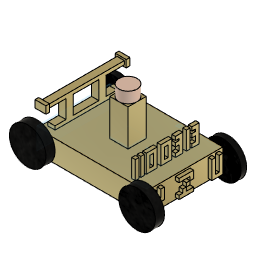
final_project_1100313 (Autodesk Fusion 360 design; units mm, degrees)
Autodesk Fusion 360 part; units mm, degrees
note: some values were not read from the file. Chosen so that the rebuilt part matches the saved one: which face or edge a step refers to; that a step has no effect; which bodies a step acts on; which pieces of a blend or face edit are solid.
(part 1 of 2)
sketch "Sketch1" plane through (0, 0, 0) normal (0, 0, 1) x (1, 0, 0)
  line L0 (150, 100) -> (-150, 100)
  line L1 (-150, 100) -> (-150, -100)
  line L2 (-150, -100) -> (150, -100)
  line L3 (150, -100) -> (150, 100)
  line L4 (150, 100) -> (-150, -100) construction
  line L5 (-150, 100) -> (150, -100) construction
  dimension "d1" = 300
  dimension "d2" = 200
  constraint horizontal L0
  constraint perpendicular L0 L1
  constraint parallel L0 L2
  constraint parallel L1 L3
  constraint coincident L4 origin
  constraint coincident L5 origin
  measures "d1" distance of L1.end L2.end
  measures "d2" distance of L0.end L1.end
extrude "Extrude1" add sketch "Sketch1" along normal blind 60 makes body 1
sketch "Sketch2" plane through (0, -100, 0) normal (0, -1, 0) x (1, 0, 0)
  line L0 (-150, 0) -> (150, 0)
  line L1 (150, 0) -> (150, 60)
  line L2 (150, 60) -> (-150, 60)
  line L3 (-150, 60) -> (-150, 0)
  circle A0 centre (-75, 25) radius 50
  circle A1 centre (75, 25) radius 50
  dimension "d5" = 100
  dimension "d6" = 100
  measures "d5" diameter of A0
  measures "d6" diameter of A1
extrude "Extrude2" add sketch "Sketch2" along normal blind 25 separate body contours L0 L2 A0 | L0 A0 | L2 A0 | L0 L2 A1 | L0 A1 | L2 A1 makes body 2 at (71.2913, -125, 8.7512) makes body 3 at (-86.1319, -125, 43.5386)
sketch "Sketch3" plane through (0, 100, 0) normal (0, 1, 0) x (-1, 0, 0)
  line L0 (-150, 0) -> (150, 0)
  line L1 (150, 0) -> (150, 60)
  line L2 (150, 60) -> (-150, 60)
  line L3 (-150, 60) -> (-150, 0)
  circle A0 centre (-75, 25) radius 50
  circle A1 centre (75, 25) radius 50
  dimension "d9" = 100
  dimension "d10" = 100
  measures "d9" diameter of A0
  measures "d10" diameter of A1
extrude "Extrude3" add sketch "Sketch3" along normal blind 25 separate body contours L0 L2 A0 | L0 A0 | L2 A0 | L0 L2 A1 | L0 A1 | L2 A1 makes body 4 at (86.1319, 125, 43.5386) makes body 5 at (-77.4632, 125, 25.3713)
move_body "Move1" bodies 1 2 3 4 5 to x (1, 0, 0) y (0, 1, 0) z (0, 0, 1) at (0, 0, 25)
sketch "Sketch4" plane through (150, 0, 0) normal (1, 0, 0) x (0, 1, 0)
  line L0 (-100, 25) -> (100, 25)
  line L1 (100, 25) -> (100, 85)
  line L2 (100, 85) -> (-100, 85)
  line L3 (-100, 85) -> (-100, 25)
  line L4 (-90, 80) -> (-80, 80)
  line L5 (-80, 80) -> (-80, 60)
  line L6 (-80, 60) -> (-90, 60)
  line L7 (-90, 60) -> (-90, 80)
  line L8 (-80, 70) -> (-60, 70)
  line L9 (-60, 70) -> (-60, 60)
  line L10 (-60, 60) -> (-80, 60)
  line L11 (-80, 60) -> (-80, 70)
  line L12 (-70, 80) -> (-60, 80)
  line L13 (-60, 80) -> (-60, 70)
  line L14 (-60, 70) -> (-70, 70)
  line L15 (-70, 70) -> (-70, 80)
  line L16 (-80, 60) -> (-70, 60)
  line L17 (-70, 60) -> (-70, 30)
  line L18 (-70, 30) -> (-80, 30)
  line L19 (-80, 30) -> (-80, 60)
  line L20 (-20, 80) -> (20, 80)
  line L21 (20, 80) -> (20, 70)
  line L22 (20, 70) -> (-20, 70)
  line L23 (-20, 70) -> (-20, 80)
  line L24 (10, 70) -> (20, 70)
  line L25 (20, 70) -> (20, 60)
  line L26 (20, 60) -> (10, 60)
  line L27 (10, 60) -> (10, 70)
  line L28 (10, 60) -> (0, 60)
  line L29 (0, 60) -> (0, 50)
  line L30 (0, 50) -> (10, 50)
  line L31 (10, 50) -> (10, 60)
  line L32 (0, 50) -> (-10, 50)
  line L33 (-10, 50) -> (-10, 40)
  line L34 (-10, 40) -> (0, 40)
  line L35 (0, 40) -> (0, 50)
  line L36 (-10, 40) -> (-20, 40)
  line L37 (-20, 40) -> (-20, 30)
  line L38 (-20, 30) -> (-10, 30)
  line L39 (-10, 30) -> (-10, 40)
  line L40 (20, 40) -> (-10, 40)
  line L41 (-10, 40) -> (-10, 30)
  line L42 (-10, 30) -> (20, 30)
  line L43 (20, 30) -> (20, 40)
  line L44 (50, 80) -> (60, 80)
  line L45 (60, 80) -> (60, 40)
  line L46 (60, 40) -> (50, 40)
  line L47 (50, 40) -> (50, 80)
  line L48 (50, 40) -> (90, 40)
  line L49 (90, 40) -> (90, 30)
  line L50 (90, 30) -> (50, 30)
  line L51 (50, 30) -> (50, 40)
  line L52 (80, 40) -> (90, 40)
  line L53 (90, 40) -> (90, 80)
  line L54 (90, 80) -> (80, 80)
  line L55 (80, 80) -> (80, 40)
  constraint horizontal L4
  constraint vertical L5
  constraint horizontal L6
  constraint vertical L7
  constraint horizontal L8
  constraint vertical L9
  constraint horizontal L10
  constraint vertical L11
  constraint midpoint L5 L8.start
  constraint horizontal L12
  constraint vertical L13
  constraint horizontal L14
  constraint vertical L15
  constraint horizontal L16
  constraint vertical L17
  constraint horizontal L18
  constraint vertical L19
  constraint horizontal L20
  constraint vertical L21
  constraint horizontal L22
  constraint vertical L23
  constraint horizontal L24
  constraint vertical L25
  constraint horizontal L26
  constraint vertical L27
  constraint coincident L22 L24.start
  constraint horizontal L28
  constraint vertical L29
  constraint horizontal L30
  constraint vertical L31
  constraint horizontal L32
  constraint vertical L33
  constraint horizontal L34
  constraint vertical L35
  constraint horizontal L36
  constraint vertical L37
  constraint horizontal L38
  constraint vertical L39
  constraint horizontal L40
  constraint vertical L41
  constraint horizontal L42
  constraint vertical L43
  constraint horizontal L44
  constraint vertical L45
  constraint horizontal L46
  constraint vertical L47
  constraint horizontal L48
  constraint vertical L49
  constraint horizontal L50
  constraint vertical L51
  constraint horizontal L52
  constraint vertical L53
  constraint horizontal L54
  constraint vertical L55
  constraint coincident L48 L52.start
sketch "Sketch5" plane through (-150, 0, 0) normal (-1, 0, 0) x (0, -1, 0)
  line L0 (-100, 25) -> (100, 25)
  line L1 (100, 25) -> (100, 85)
  line L2 (100, 85) -> (-100, 85)
  line L3 (-100, 85) -> (-100, 25)
form "Form1" [no effect]
sketch "Sketch6" plane through (0, 0, 85) normal (0, 0, 1) x (-1, 0, 0)
  line L0 (-150, 100) -> (-150, -100)
  line L1 (-150, -100) -> (150, -100)
  line L2 (150, -100) -> (150, 100)
  line L3 (150, 100) -> (-150, 100)
  line L4 (25, 25) -> (-25, 25)
  line L5 (-25, 25) -> (-25, -25)
  line L6 (-25, -25) -> (25, -25)
  line L7 (25, -25) -> (25, 25)
  line L8 (25, 25) -> (-25, -25) construction
  line L9 (-25, 25) -> (25, -25) construction
  dimension "d27" = 50
  dimension "d28" = 50
  constraint horizontal L4
  constraint perpendicular L4 L5
  constraint parallel L4 L6
  constraint parallel L5 L7
  constraint coincident L8 origin
  constraint coincident L9 origin
  measures "d27" distance of L5.end L6.end
  measures "d28" distance of L4.end L5.end
extrude "Extrude11" add sketch "Sketch6" along normal blind 100 contours L4 L5 L6 L7 bodies 1
sketch "Sketch7" plane through (0, 0, 185) normal (0, 0, 1) x (-1, 0, 0)
  line L0 (25, -25) -> (25, 25)
  line L1 (25, 25) -> (-25, 25)
  line L2 (-25, 25) -> (-25, -25)
  line L3 (-25, -25) -> (25, -25)
  circle A0 centre (0, 0) radius 25
  dimension "d31" = 50
  constraint coincident A0.centre origin
  measures "d31" diameter of A0
extrude "Extrude12" add sketch "Sketch7" along normal blind 30 separate body contours A0 makes body 6
sketch "Sketch8" plane through (-150, 0, 55) normal (-1, 0, 0) x (0, -1, 0)
  line L0 (-100, 10) -> (-80, 10)
  line L1 (-80, 10) -> (-80, -10)
  line L2 (-80, -10) -> (-100, -10)
  line L3 (-100, -10) -> (-100, 10)
  line L4 (100, 10) -> (80, 10)
  line L5 (80, 10) -> (80, -10)
  line L6 (80, -10) -> (100, -10)
  line L7 (100, -10) -> (100, 10)
  constraint horizontal L0
  constraint vertical L1
  constraint horizontal L2
  constraint vertical L3
  constraint horizontal L4
  constraint vertical L5
  constraint horizontal L6
  constraint vertical L7
sketch "Sketch9" plane through (-150, 0, 55) normal (-1, 0, 0) x (0, -1, 0)
  line L0 (-60, -10) -> (-80, -10)
  line L1 (-80, -10) -> (-80, 10)
  line L2 (-80, 10) -> (-60, 10)
  line L3 (-60, 10) -> (-60, -10)
  line L4 (-60, -10) -> (-80, 10) construction
  line L5 (-80, -10) -> (-60, 10) construction
  line L6 (80, -10) -> (60, -10)
  line L7 (60, -10) -> (60, 10)
  line L8 (60, 10) -> (80, 10)
  line L9 (80, 10) -> (80, -10)
  line L10 (80, -10) -> (60, 10) construction
  line L11 (60, -10) -> (80, 10) construction
  point P0 (-70, 0)
  point P1 (70, 0)
  constraint horizontal L0
  constraint perpendicular L0 L1
  constraint parallel L0 L2
  constraint parallel L1 L3
  constraint coincident L4 P0
  constraint coincident L5 P0
  constraint horizontal L6
  constraint perpendicular L6 L7
  constraint parallel L6 L8
  constraint parallel L7 L9
  constraint coincident L10 P1
  constraint coincident L11 P1
sketch "Sketch10" plane through (0, 0, 85) normal (0, 0, 1) x (-1, 0, 0)
  line L0 (25, -25) -> (-25, -25)
  line L1 (-25, -25) -> (-25, 25)
  line L2 (-25, 25) -> (25, 25)
  line L3 (25, 25) -> (25, -25)
  line L4 (-150, 100) -> (-150, -100)
  line L5 (-150, -100) -> (150, -100)
  line L6 (150, -100) -> (150, 100)
  line L7 (150, 100) -> (-150, 100)
  line L8 (120, 80) -> (140, 80)
  line L9 (140, 80) -> (140, -80)
  line L10 (140, -80) -> (120, -80)
  line L11 (120, -80) -> (120, 80)
  constraint horizontal L8
  constraint vertical L9
  constraint horizontal L10
  constraint vertical L11
sketch "Sketch11" plane through (0, 0, 105) normal (0, 0, 1) x (-1, 0, 0)
  line L0 (120, -80) -> (140, -80)
  line L1 (140, -80) -> (140, 80)
  line L2 (140, 80) -> (120, 80)
  line L3 (120, 80) -> (120, -80)
  line L4 (120, 40) -> (140, 40)
  line L5 (140, 40) -> (140, 20)
  line L6 (140, 20) -> (120, 20)
  line L7 (120, 20) -> (120, 40)
  line L8 (120, -20) -> (140, -20)
  line L9 (140, -20) -> (140, -40)
  line L10 (140, -40) -> (120, -40)
  line L11 (120, -40) -> (120, -20)
  constraint horizontal L4
  constraint vertical L5
  constraint horizontal L6
  constraint vertical L7
  constraint coincident L1 L5.end
  constraint coincident L3 L4.start
  constraint horizontal L8
  constraint vertical L9
  constraint horizontal L10
  constraint vertical L11
  constraint coincident L1 L9.end
  constraint coincident L3 L8.start
sketch "Sketch12" plane through (0, 0, 135) normal (0, 0, 1) x (-1, 0, 0)
  line L0 (120, 20) -> (140, 20)
  line L1 (140, 20) -> (140, 40)
  line L2 (140, 40) -> (120, 40)
  line L3 (120, 40) -> (120, 20)
  line L4 (120, 110) -> (140, 110)
  line L5 (140, 110) -> (140, -110)
  line L6 (140, -110) -> (120, -110)
  line L7 (120, -110) -> (120, 110)
  constraint horizontal L4
  constraint vertical L5
  constraint horizontal L6
  constraint vertical L7
sketch "Sketch13" plane through (0, 110, 0) normal (0, 1, 0) x (-1, 0, 0)
  line L0 (120, 135) -> (140, 135)
  line L1 (140, 135) -> (140, 155)
  line L2 (140, 155) -> (120, 155)
  line L3 (120, 155) -> (120, 135)
  line L4 (150, 135) -> (110, 135)
  line L5 (110, 135) -> (110, 155)
  line L6 (110, 155) -> (150, 155)
  line L7 (150, 155) -> (150, 135)
  line L8 (150, 135) -> (110, 155) construction
  line L9 (110, 135) -> (150, 155) construction
  point P0 (130, 145)
  dimension "d44" = 40
  dimension "d45" = 20
  constraint horizontal L4
  constraint perpendicular L4 L5
  constraint parallel L4 L6
  constraint parallel L5 L7
  constraint coincident L8 P0
  constraint coincident L9 P0
  measures "d44" distance of L5.end L6.end
  measures "d45" distance of L4.end L5.end
sketch "Sketch14" plane through (0, -110, 0) normal (0, -1, 0) x (1, 0, 0)
  line L0 (-140, 135) -> (-120, 135)
  line L1 (-120, 135) -> (-120, 155)
  line L2 (-120, 155) -> (-140, 155)
  line L3 (-140, 155) -> (-140, 135)
  line L4 (-109.8517, 135) -> (-149.8517, 135)
  line L5 (-149.8517, 135) -> (-149.8517, 155)
  line L6 (-149.8517, 155) -> (-109.8517, 155)
  line L7 (-109.8517, 155) -> (-109.8517, 135)
  line L8 (-109.8517, 135) -> (-149.8517, 155) construction
  line L9 (-149.8517, 135) -> (-109.8517, 155) construction
  point P0 (-129.8517, 145)
  dimension "d48" = 40
  dimension "d49" = 20
  constraint horizontal L4
  constraint perpendicular L4 L5
  constraint parallel L4 L6
  constraint parallel L5 L7
  constraint coincident L8 P0
  constraint coincident L9 P0
  measures "d48" distance of L5.end L6.end
  measures "d49" distance of L4.end L5.end
sketch "Sketch15" plane through (0, 0, 85) normal (0, 0, 1) x (-1, 0, 0)
  line L0 (25, -25) -> (-25, -25)
  line L1 (-25, -25) -> (-25, 25)
  line L2 (-25, 25) -> (25, 25)
  line L3 (25, 25) -> (25, -25)
  line L4 (-150, 100) -> (-150, -100)
  line L5 (-150, -100) -> (150, -100)
  line L6 (150, -100) -> (150, 100)
  line L7 (150, 100) -> (-150, 100)
sketch "Sketch16" plane through (0, 0, 85) normal (0, 0, 1) x (-1, 0, 0)
  line L0 (-100, 90) -> (-90, 90)
  line L1 (-90, 90) -> (-90, 80)
  line L2 (-90, 80) -> (-100, 80)
  line L3 (-100, 80) -> (-100, 90)
  constraint horizontal L0
  constraint vertical L1
  constraint horizontal L2
  constraint vertical L3
sketch "Sketch17" plane through (0, 0, 85) normal (0, 0, 1) x (1, 0, 0)
  line L0 (100, -70) -> (90, -70)
  line L1 (90, -70) -> (90, -60)
  line L2 (90, -60) -> (100, -60)
  line L3 (100, -60) -> (100, -70)
  constraint horizontal L0
  constraint vertical L1
  constraint horizontal L2
  constraint vertical L3
sketch "Sketch18" plane through (0, 0, 85) normal (0, 0, 1) x (-1, 0, 0)
  line L0 (-100, 50) -> (-90, 50)
  line L1 (-90, 50) -> (-90, 20)
  line L2 (-90, 20) -> (-100, 20)
  line L3 (-100, 20) -> (-100, 50)
  constraint horizontal L0
  constraint vertical L1
  constraint horizontal L2
  constraint vertical L3
sketch "Sketch19" plane through (0, 0, 95) normal (0, 0, 1) x (-1, 0, 0)
  line L0 (-100, 20) -> (-90, 20)
  line L1 (-90, 20) -> (-90, 50)
  line L2 (-90, 50) -> (-100, 50)
  line L3 (-100, 50) -> (-100, 20)
  line L4 (-90, 20) -> (-100, 20)
  line L5 (-100, 20) -> (-100, 30)
  line L6 (-100, 30) -> (-90, 30)
  line L7 (-90, 30) -> (-90, 20)
  line L8 (-90, 40) -> (-100, 40)
  line L9 (-100, 40) -> (-100, 50)
  line L10 (-100, 50) -> (-90, 50)
  line L11 (-90, 50) -> (-90, 40)
  constraint horizontal L4
  constraint vertical L5
  constraint horizontal L6
  constraint vertical L7
  constraint coincident L3 L5.end
  constraint coincident L0.end L1.start
  constraint horizontal L8
  constraint vertical L9
  constraint horizontal L10
  constraint vertical L11
  constraint coincident L3 L2.end
sketch "Sketch20" plane through (0, 0, 95) normal (0, 0, 1) x (-1, 0, 0)
sketch "Sketch21" plane through (0, 0, 125) normal (0, 0, 1) x (-1, 0, 0)
  line L0 (-90, 30) -> (-100, 30)
  line L1 (-100, 30) -> (-100, 20)
  line L2 (-100, 20) -> (-90, 20)
  line L3 (-90, 20) -> (-90, 30)
  line L4 (-90, 20) -> (-100, 20)
  line L5 (-100, 20) -> (-100, 50)
  line L6 (-100, 50) -> (-90, 50)
  line L7 (-90, 50) -> (-90, 20)
  constraint horizontal L4
  constraint vertical L5
  constraint horizontal L6
  constraint vertical L7
  constraint coincident L2.end L3.start
sketch "Sketch22" plane through (0, 0, 85) normal (0, 0, 1) x (-1, 0, 0)
  line L0 (-100, 10) -> (-90, 10)
  line L1 (-90, 10) -> (-90, -20)
  line L2 (-90, -20) -> (-100, -20)
  line L3 (-100, -20) -> (-100, 10)
  constraint horizontal L0
  constraint vertical L1
  constraint horizontal L2
  constraint vertical L3
sketch "Sketch23" plane through (0, 0, 95) normal (0, 0, 1) x (-1, 0, 0)
  line L0 (-100, -20) -> (-90, -20)
  line L1 (-90, -20) -> (-90, 10)
  line L2 (-90, 10) -> (-100, 10)
  line L3 (-100, 10) -> (-100, -20)
  line L4 (-90, -20) -> (-100, -20)
  line L5 (-100, -20) -> (-100, -10)
  line L6 (-100, -10) -> (-90, -10)
  line L7 (-90, -10) -> (-90, -20)
  line L8 (-90, 0) -> (-100, 0)
  line L9 (-100, 0) -> (-100, 10)
  line L10 (-100, 10) -> (-90, 10)
  line L11 (-90, 10) -> (-90, 0)
  constraint horizontal L4
  constraint vertical L5
  constraint horizontal L6
  constraint vertical L7
  constraint coincident L3 L5.end
  constraint coincident L0.end L1.start
  constraint horizontal L8
  constraint vertical L9
  constraint horizontal L10
  constraint vertical L11
  constraint coincident L2.end L3.start
  constraint coincident L1 L8.start
sketch "Sketch24" plane through (0, 0, 125) normal (0, 0, 1) x (-1, 0, 0)
  line L0 (-90, -10) -> (-100, -10)
  line L1 (-100, -10) -> (-100, -20)
  line L2 (-100, -20) -> (-90, -20)
  line L3 (-90, -20) -> (-90, -10)
  line L4 (-90, -20) -> (-100, -20)
  line L5 (-100, -20) -> (-100, 10)
  line L6 (-100, 10) -> (-90, 10)
  line L7 (-90, 10) -> (-90, -20)
  constraint horizontal L4
  constraint vertical L5
  constraint horizontal L6
  constraint vertical L7
  constraint coincident L2.end L3.start
sketch "Sketch25" plane through (0, 0, 85) normal (0, 0, 1) x (-1, 0, 0)
  line L0 (-100, -30) -> (-90, -30)
  line L1 (-90, -30) -> (-90, -50)
  line L2 (-90, -50) -> (-100, -50)
  line L3 (-100, -50) -> (-100, -30)
  constraint horizontal L0
  constraint vertical L1
  constraint horizontal L2
  constraint vertical L3
sketch "Sketch26" plane through (0, 0, 95) normal (0, 0, 1) x (-1, 0, 0)
  line L0 (-100, -50) -> (-90, -50)
  line L1 (-90, -50) -> (-90, -30)
  line L2 (-90, -30) -> (-100, -30)
  line L3 (-100, -30) -> (-100, -50)
  line L4 (-90, -50) -> (-100, -50)
  line L5 (-100, -50) -> (-100, -40)
  line L6 (-100, -40) -> (-90, -40)
  line L7 (-90, -40) -> (-90, -50)
  constraint horizontal L4
  constraint vertical L5
  constraint horizontal L6
  constraint vertical L7
  constraint midpoint L3 L5.end
  constraint coincident L0.end L1.start
sketch "Sketch27" plane through (0, 40, 0) normal (0, -1, 0) x (1, 0, 0)
  line L0 (100, 95) -> (100, 135)
  line L1 (100, 135) -> (90, 135)
  line L2 (90, 135) -> (90, 95)
  line L3 (100, 120) -> (90, 120)
  line L4 (90, 120) -> (90, 110)
  line L5 (90, 110) -> (100, 110)
  line L6 (100, 110) -> (100, 120)
  line L7 (90, 95) -> (100, 95)
  constraint horizontal L3
  constraint vertical L4
  constraint horizontal L5
  constraint vertical L6
  constraint coincident L2 L4.end
  constraint coincident L0 L3.start
sketch "Sketch28" plane through (0, 0, 135) normal (0, 0, 1) x (-1, 0, 0)
  line L0 (-90, -40) -> (-100, -40)
  line L1 (-100, -40) -> (-100, -50)
  line L2 (-100, -50) -> (-90, -50)
  line L3 (-90, -50) -> (-90, -40)
sketch "Sketch29" plane through (0, 40, 0) normal (0, -1, 0) x (1, 0, 0)
  line L0 (90, 120) -> (100, 120)
  line L1 (100, 120) -> (100, 135)
  line L2 (100, 135) -> (90, 135)
  line L3 (90, 135) -> (90, 120)
  line L4 (90, 135) -> (100, 135)
  line L5 (100, 135) -> (100, 125)
  line L6 (100, 125) -> (90, 125)
  line L7 (90, 125) -> (90, 135)
  dimension "d74" = 10
  dimension "d75" = 10
  constraint horizontal L4
  constraint vertical L5
  constraint horizontal L6
  constraint vertical L7
  constraint coincident L2.end L3.start
  measures "d74" distance of L2.end L1.end
  measures "d75" distance of L2.end L6.end
sketch "Sketch30" plane through (0, 0, 85) normal (0, 0, 1) x (1, 0, 0)
  line L0 (100, 60) -> (90, 60)
  line L1 (90, 60) -> (90, 70)
  line L2 (90, 70) -> (100, 70)
  line L3 (100, 70) -> (100, 60)
  constraint horizontal L0
  constraint vertical L1
  constraint horizontal L2
  constraint vertical L3
sketch "Sketch31" plane through (0, 0, 85) normal (0, 0, 1) x (-1, 0, 0)
  line L0 (-90, -100) -> (-100, -100)
  line L1 (-100, -100) -> (-100, -80)
  line L2 (-100, -80) -> (-90, -80)
  line L3 (-90, -80) -> (-90, -100)
  constraint horizontal L0
  constraint vertical L1
  constraint horizontal L2
  constraint vertical L3
extrude "Extrude33" add sketch "Sketch31" along normal blind 10 separate body makes body 7
sketch "Sketch32" plane through (0, 0, 95) normal (0, 0, 1) x (-1, 0, 0)
  line L0 (-90, -80) -> (-100, -80)
  line L1 (-100, -80) -> (-100, -100)
  line L2 (-100, -100) -> (-90, -100)
  line L3 (-90, -100) -> (-90, -80)
extrude "Extrude34" add 1 faces at (87.958, 125, 70.2329) along direction (0, 1, 0) blind 10 on bodies 4 bodies 4
extrude "Extrude35" add 1 faces at (-77.4632, 125, 50.3713) along direction (0, 1, 0) blind 10 on bodies 5 bodies 5
extrude "Extrude36" cut 1 faces at (79.0441, 100, 62.5152) along direction (0, 1, 0) blind 10 on bodies 4 bodies 4
extrude "Extrude37" cut 1 faces at (-61.4482, 100, 47.516) along direction (0, 1, 0) blind 10 on bodies 5 bodies 5
extrude "Extrude38" add 1 faces at (50, 100, 45) along direction (0, 1, 0) blind 10 separate body on bodies 1 makes body 8
extrude "Extrude39" cut 1 faces at (50, 110, 45) along direction (0, -1, 0) blind 10 on bodies 8 bodies 8
extrude "Extrude40" cut 1 faces at (79.0441, 110, 62.5152) along direction (0, 1, 0) blind 10 on bodies 4 bodies 4
extrude "Extrude41" cut 1 faces at (-61.4482, 110, 47.516) along direction (0, 1, 0) blind 10 on bodies 5 bodies 5
extrude "Extrude42" add 1 faces at (50, 100, 45) along direction (0, 1, 0) blind 10 on bodies 1 bodies 2 3 1 6 4 5 7
move_body "Move2" bodies 4 to x (1, 0, 0) y (0, 1, 0) z (0, 0, 1) at (0, -10, 0)
move_body "Move3" bodies 5 to x (1, 0, 0) y (0, 1, 0) z (0, 0, 1) at (0, -10, 0)
sketch "Sketch33" plane through (0, 0, 95) normal (0, 0, 1) x (-1, 0, 0)
delete_face "DeleteFace1" 1 faces at (100, 93.3333, 88.3333) on bodies 1
sketch "Sketch34" plane through (0, 0, 85) normal (0, 0, 1) x (-1, 0, 0)
  line L0 (-100, -80) -> (-90, -80)
  line L1 (-90, -80) -> (-90, -100)
  line L2 (-90, -100) -> (-100, -100)
  line L3 (-100, -100) -> (-100, -80)
  constraint horizontal L0
  constraint vertical L1
  constraint horizontal L2
  constraint vertical L3
sketch "Sketch35" plane through (0, 0, 95) normal (0, 0, 1) x (-1, 0, 0)
  line L0 (-100, -90) -> (-90, -90)
  line L1 (-90, -90) -> (-90, -100)
  line L2 (-90, -100) -> (-100, -100)
  line L3 (-100, -100) -> (-100, -90)
  constraint horizontal L0
  constraint vertical L1
  constraint horizontal L2
  constraint vertical L3
sketch "Sketch36" plane through (0, 90, 0) normal (0, -1, 0) x (1, 0, 0)
  line L0 (100, 95) -> (100, 135)
  line L1 (100, 135) -> (90, 135)
  line L2 (90, 135) -> (90, 95)
  line L3 (90, 135) -> (100, 135)
  line L4 (100, 135) -> (100, 125)
  line L5 (100, 125) -> (90, 125)
  line L6 (90, 125) -> (90, 135)
  line L7 (100, 120) -> (90, 120)
  line L8 (90, 120) -> (90, 110)
  line L9 (90, 110) -> (100, 110)
  line L10 (100, 110) -> (100, 120)
  line L11 (90, 95) -> (100, 95)
  dimension "d104" = 10
  constraint horizontal L3
  constraint vertical L4
  constraint horizontal L5
  constraint vertical L6
  constraint coincident L1.end L2.start
  constraint horizontal L7
  constraint vertical L8
  constraint horizontal L9
  constraint vertical L10
  constraint coincident L2 L8.end
  constraint coincident L0 L7.start
  measures "d104" distance of L1.end L5.end
extrude "Extrude46" cut 1 faces at (150, 40, 65) along direction (1, 0, 0) blind 10 on bodies 1 bodies 1
sketch "Sketch37" plane through (-150, 0, 0) normal (-1, 0, 0) x (0, -1, 0)
  line L0 (100, 85) -> (-110, 85)
  line L1 (-110, 85) -> (-110, 25)
  line L2 (-110, 25) -> (100, 25)
  line L3 (100, 25) -> (100, 85)
  line L4 (-110, 65.7658) -> (-90, 65.7658)
  line L5 (-90, 65.7658) -> (-90, 45.7658)
  line L6 (-90, 45.7658) -> (-110, 45.7658)
  line L7 (-110, 45.7658) -> (-110, 65.7658)
  dimension "d109" = 20
  dimension "d110" = 20
  constraint horizontal L4
  constraint vertical L5
  constraint horizontal L6
  constraint vertical L7
  constraint coincident L1 L4.start
  measures "d109" distance of L4.start L4.end
  measures "d110" distance of L4.start L6.end
sketch "Sketch38" plane through (-150, 0, 0) normal (-1, 0, 0) x (0, -1, 0)
  line L0 (-90.1315, 65.7658) -> (-70.1315, 65.7658)
  line L1 (-70.1315, 65.7658) -> (-70.1315, 45.7658)
  line L2 (-70.1315, 45.7658) -> (-90.1315, 45.7658)
  line L3 (-90.1315, 45.7658) -> (-90.1315, 65.7658)
  dimension "d115" = 20
  dimension "d116" = 20
  constraint horizontal L0
  constraint vertical L1
  constraint horizontal L2
  constraint vertical L3
  measures "d115" distance of L0.start L0.end
  measures "d116" distance of L0.start L2.end
sketch "Sketch39" plane through (-150, 0, 0) normal (-1, 0, 0) x (0, -1, 0)
  line L0 (80.2127, 64.9033) -> (60.2127, 64.9033)
  line L1 (60.2127, 64.9033) -> (60.2127, 44.9033)
  line L2 (60.2127, 44.9033) -> (80.2127, 44.9033)
  line L3 (80.2127, 44.9033) -> (80.2127, 64.9033)
  dimension "d119" = 20
  dimension "d120" = 20
  constraint horizontal L0
  constraint vertical L1
  constraint horizontal L2
  constraint vertical L3
  measures "d119" distance of L0.start L0.end
  measures "d120" distance of L0.start L2.end
copy_body "Body->Comp2" bodies 2 removing the originals makes body 9 in component "right_wheel1"
copy_body "Body->Comp3" bodies 3 removing the originals makes body 10 in component "right_wheel2"
copy_body "Body->Comp4" bodies 4 removing the originals makes body 11 in component "left_wheel1"
copy_body "Body->Comp5" bodies 5 removing the originals makes body 12 in component "left_wheel2"
copy_body "Body->Comp9" bodies 6 removing the originals makes body 13 in component "lidar"
sketch "Sketch40" plane through (150, 0, 0) normal (1, 0, 0) x (0, 1, 0)
  line L0 (-100, 25) -> (110, 25)
  line L1 (110, 25) -> (110, 85)
  line L2 (110, 85) -> (-100, 85)
  line L3 (-100, 85) -> (-100, 25)
  line L4 (-90, 80) -> (-80, 80)
  line L5 (-80, 80) -> (-80, 50)
  line L6 (-80, 50) -> (-90, 50)
  line L7 (-90, 50) -> (-90, 80)
  line L8 (-80, 60) -> (-60, 60)
  line L9 (-60, 60) -> (-60, 50)
  line L10 (-60, 50) -> (-80, 50)
  line L11 (-80, 50) -> (-80, 60)
  line L12 (-60, 60) -> (-70, 60)
  line L13 (-70, 60) -> (-70, 80)
  line L14 (-70, 80) -> (-60, 80)
  line L15 (-60, 80) -> (-60, 60)
  line L16 (-70, 50) -> (-80, 50)
  line L17 (-80, 50) -> (-80, 25.2282)
  line L18 (-80, 25.2282) -> (-70, 25.2282)
  line L19 (-70, 25.2282) -> (-70, 50)
  constraint horizontal L4
  constraint vertical L5
  constraint horizontal L6
  constraint vertical L7
  constraint horizontal L8
  constraint vertical L9
  constraint horizontal L10
  constraint vertical L11
  constraint coincident L5 L8.start
  constraint horizontal L12
  constraint vertical L13
  constraint horizontal L14
  constraint vertical L15
  constraint horizontal L16
  constraint vertical L17
  constraint horizontal L18
  constraint vertical L19
  constraint midpoint L10 L16.start
sketch "Sketch41" plane through (150, 0, 0) normal (1, 0, 0) x (0, 1, 0)
  line L0 (-80, 50) -> (-90, 50)
  line L1 (-90, 50) -> (-90, 80)
  line L2 (-90, 80) -> (-80, 80)
  line L3 (-80, 80) -> (-80, 60)
  line L4 (-80, 60) -> (-70, 60)
  line L5 (-70, 60) -> (-70, 80)
  line L6 (-70, 80) -> (-60, 80)
  line L7 (-60, 80) -> (-60, 50)
  line L8 (-60, 50) -> (-70, 50)
  line L9 (-70, 50) -> (-70, 25.2282)
  line L10 (-70, 25.2282) -> (-80, 25.2282)
  line L11 (-80, 25.2282) -> (-80, 50)
  line L12 (-100, 25) -> (110, 25)
  line L13 (110, 25) -> (110, 85)
  line L14 (110, 85) -> (-100, 85)
  line L15 (-100, 85) -> (-100, 25)
  line L16 (-20, 80) -> (20, 80)
  line L17 (20, 80) -> (20, 70)
  line L18 (20, 70) -> (-20, 70)
  line L19 (-20, 70) -> (-20, 80)
  line L20 (20, 70) -> (10, 70)
  line L21 (10, 70) -> (10, 60)
  line L22 (10, 60) -> (20, 60)
  line L23 (20, 60) -> (20, 70)
  line L24 (10, 60) -> (0, 60)
  line L25 (0, 60) -> (0, 50)
  line L26 (0, 50) -> (10, 50)
  line L27 (10, 50) -> (10, 60)
  line L28 (0, 50) -> (-10, 50)
  line L29 (-10, 50) -> (-10, 40)
  line L30 (-10, 40) -> (0, 40)
  line L31 (0, 40) -> (0, 50)
  line L32 (-20, 40) -> (20, 40)
  line L33 (20, 40) -> (20, 30)
  line L34 (20, 30) -> (-20, 30)
  line L35 (-20, 30) -> (-20, 40)
  constraint horizontal L16
  constraint vertical L17
  constraint horizontal L18
  constraint vertical L19
  constraint horizontal L20
  constraint vertical L21
  constraint horizontal L22
  constraint vertical L23
  constraint horizontal L24
  constraint vertical L25
  constraint horizontal L26
  constraint vertical L27
  constraint horizontal L28
  constraint vertical L29
  constraint horizontal L30
  constraint vertical L31
  constraint horizontal L32
  constraint vertical L33
  constraint horizontal L34
  constraint vertical L35
sketch "Sketch42" plane through (160, 0, 0) normal (1, 0, 0) x (0, 1, 0)
  line L0 (0, 40) -> (0, 50)
  line L1 (0, 50) -> (-10, 50)
  line L2 (-10, 50) -> (-10, 40)
  line L3 (-10, 40) -> (-20, 40)
  line L4 (-20, 40) -> (-20, 30)
  line L5 (-20, 30) -> (20, 30)
  line L6 (20, 30) -> (20, 40)
  line L7 (20, 40) -> (0, 40)
  line L8 (70, 80) -> (80, 80)
  line L9 (80, 80) -> (80, 30)
  line L10 (80, 30) -> (70, 30)
  line L11 (70, 30) -> (70, 80)
  line L12 (80, 40) -> (90, 40)
  line L13 (90, 40) -> (90, 30)
  line L14 (90, 30) -> (80, 30)
  line L15 (80, 30) -> (80, 40)
  line L16 (90, 80) -> (100, 80)
  line L17 (100, 80) -> (100, 30)
  line L18 (100, 30) -> (90, 30)
  line L19 (90, 30) -> (90, 80)
  constraint horizontal L8
  constraint vertical L9
  constraint horizontal L10
  constraint vertical L11
  constraint horizontal L12
  constraint vertical L13
  constraint horizontal L14
  constraint vertical L15
  constraint coincident L9 L12.start
  constraint horizontal L16
  constraint vertical L17
  constraint horizontal L18
  constraint vertical L19
sketch "Sketch43" plane through (0, 0, 85) normal (0, 0, 1) x (1, 0, 0)
  line L0 (100, -90) -> (90, -90)
  line L1 (90, -90) -> (90, -80)
  line L2 (90, -80) -> (100, -80)
  line L3 (100, -80) -> (100, -90)
  constraint horizontal L0
  constraint vertical L1
  constraint horizontal L2
  constraint vertical L3
sketch "Sketch44" plane through (0, 0, 85) normal (0, 0, 1) x (1, 0, 0)
  line L0 (100, -70) -> (90, -70)
  line L1 (90, -70) -> (90, -60)
  line L2 (90, -60) -> (100, -60)
  line L3 (100, -60) -> (100, -70)
  constraint horizontal L0
  constraint vertical L1
  constraint horizontal L2
  constraint vertical L3
sketch "Sketch45" plane through (0, 0, 85) normal (0, 0, 1) x (1, 0, 0)
  line L0 (100, -50) -> (90, -50)
  line L1 (90, -50) -> (90, -20)
  line L2 (90, -20) -> (100, -20)
  line L3 (100, -20) -> (100, -50)
  constraint horizontal L0
  constraint vertical L1
  constraint horizontal L2
  constraint vertical L3
sketch "Sketch46" plane through (0, 0, 95) normal (0, 0, 1) x (-1, 0, 0)
  line L0 (-100, 20) -> (-90, 20)
  line L1 (-90, 20) -> (-90, 50)
  line L2 (-90, 50) -> (-100, 50)
  line L3 (-100, 50) -> (-100, 20)
  line L4 (-90, 40) -> (-100, 40)
  line L5 (-100, 40) -> (-100, 50)
  line L6 (-100, 50) -> (-90, 50)
  line L7 (-90, 50) -> (-90, 40)
  line L8 (-90, 20) -> (-100, 20)
  line L9 (-100, 20) -> (-100, 30)
  line L10 (-100, 30) -> (-90, 30)
  line L11 (-90, 30) -> (-90, 20)
  constraint horizontal L4
  constraint vertical L5
  constraint horizontal L6
  constraint vertical L7
  constraint coincident L1 L4.start
  constraint horizontal L8
  constraint vertical L9
  constraint horizontal L10
  constraint vertical L11
  constraint coincident L0.end L1.start
sketch "Sketch47" plane through (0, 0, 125) normal (0, 0, 1) x (-1, 0, 0)
  line L0 (-90, 30) -> (-100, 30)
  line L1 (-100, 30) -> (-100, 20)
  line L2 (-100, 20) -> (-90, 20)
  line L3 (-90, 20) -> (-90, 30)
  line L4 (-100, 50) -> (-90, 50)
  line L5 (-90, 50) -> (-90, 20)
  line L6 (-90, 20) -> (-100, 20)
  line L7 (-100, 20) -> (-100, 50)
  constraint horizontal L4
  constraint vertical L5
  constraint horizontal L6
  constraint vertical L7
  constraint coincident L2.end L3.start
sketch "Sketch48" plane through (0, 0, 85) normal (0, 0, 1) x (-1, 0, 0)
  line L0 (-100, 10) -> (-90, 10)
  line L1 (-90, 10) -> (-90, -20)
  line L2 (-90, -20) -> (-100, -20)
  line L3 (-100, -20) -> (-100, 10)
  constraint horizontal L0
  constraint vertical L1
  constraint horizontal L2
  constraint vertical L3
sketch "Sketch49" plane through (0, 0, 95) normal (0, 0, 1) x (-1, 0, 0)
  line L0 (-100, -20) -> (-90, -20)
  line L1 (-90, -20) -> (-90, 10)
  line L2 (-90, 10) -> (-100, 10)
  line L3 (-100, 10) -> (-100, -20)
  line L4 (-100, 10) -> (-90, 10)
  line L5 (-90, 10) -> (-90, 0)
  line L6 (-90, 0) -> (-100, 0)
  line L7 (-100, 0) -> (-100, 10)
  line L8 (-100, -10) -> (-90, -10)
  line L9 (-90, -10) -> (-90, -20)
  line L10 (-90, -20) -> (-100, -20)
  line L11 (-100, -20) -> (-100, -10)
  constraint horizontal L4
  constraint vertical L5
  constraint horizontal L6
  constraint vertical L7
  constraint coincident L2.end L3.start
  constraint horizontal L8
  constraint vertical L9
  constraint horizontal L10
  constraint vertical L11
  constraint coincident L3 L8.start
sketch "Sketch50" plane through (0, 0, 125) normal (0, 0, 1) x (-1, 0, 0)
  line L0 (-100, 0) -> (-90, 0)
  line L1 (-90, 0) -> (-90, 10)
  line L2 (-90, 10) -> (-100, 10)
  line L3 (-100, 10) -> (-100, 0)
  line L4 (-100, 10) -> (-90, 10)
  line L5 (-90, 10) -> (-90, -20)
  line L6 (-90, -20) -> (-100, -20)
  line L7 (-100, -20) -> (-100, 10)
  constraint horizontal L4
  constraint vertical L5
  constraint horizontal L6
  constraint vertical L7
  constraint coincident L2.end L3.start
sketch "Sketch51" plane through (0, 0, 85) normal (0, 0, 1) x (-1, 0, 0)
  line L0 (-100, -30) -> (-90, -30)
  line L1 (-90, -30) -> (-90, -50)
  line L2 (-90, -50) -> (-100, -50)
  line L3 (-100, -50) -> (-100, -30)
  constraint horizontal L0
  constraint vertical L1
  constraint horizontal L2
  constraint vertical L3
sketch "Sketch52" plane through (0, 0, 95) normal (0, 0, 1) x (-1, 0, 0)
  line L0 (-100, -50) -> (-90, -50)
  line L1 (-90, -50) -> (-90, -30)
  line L2 (-90, -30) -> (-100, -30)
  line L3 (-100, -30) -> (-100, -50)
  line L4 (-100, -40) -> (-90, -40)
  line L5 (-90, -40) -> (-90, -50)
  line L6 (-90, -50) -> (-100, -50)
  line L7 (-100, -50) -> (-100, -40)
  constraint horizontal L4
  constraint vertical L5
  constraint horizontal L6
  constraint vertical L7
  constraint coincident L0.end L1.start
  constraint midpoint L3 L4.start
sketch "Sketch53" plane through (0, 40, 0) normal (0, -1, 0) x (1, 0, 0)
  line L0 (90, 95) -> (100, 95)
  line L1 (100, 95) -> (100, 135)
  line L2 (100, 135) -> (90, 135)
  line L3 (90, 135) -> (90, 95)
  line L4 (100, 120) -> (90, 120)
  line L5 (90, 120) -> (90, 110)
  line L6 (90, 110) -> (100, 110)
  line L7 (100, 110) -> (100, 120)
  constraint horizontal L4
  constraint vertical L5
  constraint horizontal L6
  constraint vertical L7
  constraint coincident L3 L5.end
  constraint coincident L1 L4.start
sketch "Sketch54" plane through (0, 40, 0) normal (0, -1, 0) x (1, 0, 0)
  line L0 (90, 120) -> (100, 120)
  line L1 (100, 120) -> (100, 135)
  line L2 (100, 135) -> (90, 135)
  line L3 (90, 135) -> (90, 120)
  line L4 (100, 135) -> (90, 135)
  line L5 (90, 135) -> (90, 125)
  line L6 (90, 125) -> (100, 125)
  line L7 (100, 125) -> (100, 135)
  dimension "d177" = 10
  dimension "d178" = 10
  constraint horizontal L4
  constraint vertical L5
  constraint horizontal L6
  constraint vertical L7
  constraint coincident L1.end L2.start
  measures "d177" distance of L1.end L2.end
  measures "d178" distance of L1.end L6.end
sketch "Sketch55" plane through (0, 0, 85) normal (0, 0, 1) x (-1, 0, 0)
  line L0 (-90, -60) -> (-100, -60)
  line L1 (-100, -60) -> (-100, -70)
  line L2 (-100, -70) -> (-90, -70)
  line L3 (-90, -70) -> (-90, -60)
  constraint horizontal L0
  constraint vertical L1
  constraint horizontal L2
  constraint vertical L3
sketch "Sketch56" plane through (0, 0, 95) normal (0, 0, 1) x (-1, 0, 0)
sketch "Sketch57" plane through (0, 0, 0) normal (1, 0, 0) x (0, 1, 0)
sketch "Sketch58" plane through (0, 0, 85) normal (0, 0, 1) x (-1, 0, 0)
  line L0 (-100, -80) -> (-90, -80)
  line L1 (-90, -80) -> (-90, -100)
  line L2 (-90, -100) -> (-100, -100)
  line L3 (-100, -100) -> (-100, -80)
  constraint horizontal L0
  constraint vertical L1
  constraint horizontal L2
  constraint vertical L3
sketch "Sketch59" plane through (0, 0, 95) normal (0, 0, 1) x (-1, 0, 0)
  line L0 (-100, -90) -> (-90, -90)
  line L1 (-90, -90) -> (-90, -100)
  line L2 (-90, -100) -> (-100, -100)
  line L3 (-100, -100) -> (-100, -90)
  constraint horizontal L0
  constraint vertical L1
  constraint horizontal L2
  constraint vertical L3
sketch "Sketch60" plane through (0, 90, 0) normal (0, -1, 0) x (1, 0, 0)
  line L0 (90, 95) -> (100, 95)
  line L1 (100, 95) -> (100, 135)
  line L2 (100, 135) -> (90, 135)
  line L3 (90, 135) -> (90, 95)
  line L4 (100, 120) -> (90, 120)
  line L5 (90, 120) -> (90, 110)
  line L6 (90, 110) -> (100, 110)
  line L7 (100, 110) -> (100, 120)
  constraint horizontal L4
  constraint vertical L5
  constraint horizontal L6
  constraint vertical L7
  constraint coincident L1 L4.start
sketch "Sketch61" plane through (0, 90, 0) normal (0, -1, 0) x (1, 0, 0)
  line L0 (90, 120) -> (100, 120)
  line L1 (100, 120) -> (100, 135)
  line L2 (100, 135) -> (90, 135)
  line L3 (90, 135) -> (90, 120)
  line L4 (100, 135) -> (90, 135)
  line L5 (90, 135) -> (90, 127.5)
  line L6 (90, 127.5) -> (100, 127.5)
  line L7 (100, 127.5) -> (100, 135)
  constraint horizontal L4
  constraint vertical L5
  constraint horizontal L6
  constraint vertical L7
  constraint midpoint L3 L5.end
  constraint coincident L1.end L2.start
sketch "Sketch62" plane through (150, 0, 0) normal (1, 0, 0) x (0, 1, 0)
  line L0 (-80, 50) -> (-90, 50)
  line L1 (-90, 50) -> (-90, 80)
  line L2 (-90, 80) -> (-80, 80)
  line L3 (-80, 80) -> (-80, 60)
  line L4 (-80, 60) -> (-70, 60)
  line L5 (-70, 60) -> (-70, 80)
  line L6 (-70, 80) -> (-60, 80)
  line L7 (-60, 80) -> (-60, 50)
  line L8 (-60, 50) -> (-70, 50)
  line L9 (-70, 50) -> (-70, 25.2282)
  line L10 (-70, 25.2282) -> (-80, 25.2282)
  line L11 (-80, 25.2282) -> (-80, 50)
  line L12 (-100, 25) -> (110, 25)
  line L13 (110, 25) -> (110, 85)
  line L14 (110, 85) -> (-100, 85)
  line L15 (-100, 85) -> (-100, 25)
sketch "Sketch63" plane through (-150, 0, 0) normal (-1, 0, 0) x (0, -1, 0)
sketch "Sketch64" plane through (150, 5, 55) normal (1, 0, 0) x (0, 1, 0)
  line L0 (90, 20) -> (80, 20)
  line L1 (80, 20) -> (80, -20)
  line L2 (80, -20) -> (90, -20)
  line L3 (90, -20) -> (90, 20)
  line L4 (70, 20) -> (60, 20)
  line L5 (60, 20) -> (60, -20)
  line L6 (60, -20) -> (70, -20)
  line L7 (70, -20) -> (70, 20)
  line L8 (80, -10) -> (70, -10)
  line L9 (70, -10) -> (70, -20)
  line L10 (70, -20) -> (80, -20)
  line L11 (80, -20) -> (80, -10)
  constraint horizontal L0
  constraint vertical L1
  constraint horizontal L2
  constraint vertical L3
  constraint horizontal L4
  constraint vertical L5
  constraint horizontal L6
  constraint vertical L7
  constraint horizontal L8
  constraint vertical L9
  constraint horizontal L10
  constraint vertical L11
  constraint coincident L1 L8.start
sketch "Sketch65" plane through (150, 0, 0) normal (1, 0, 0) x (0, 1, 0)
sketch "Sketch66" plane through (150, 5, 55) normal (1, 0, 0) x (0, 1, 0)
  line L0 (-20.1825, 24.646) -> (19.8175, 24.646)
  line L1 (19.8175, 24.646) -> (19.8175, 14.646)
  line L2 (19.8175, 14.646) -> (-20.1825, 14.646)
  line L3 (-20.1825, 14.646) -> (-20.1825, 24.646)
  line L4 (19.8175, 14.646) -> (9.8175, 14.646)
  line L5 (9.8175, 14.646) -> (9.8175, 4.646)
  line L6 (9.8175, 4.646) -> (19.8175, 4.646)
  line L7 (19.8175, 4.646) -> (19.8175, 14.646)
  line L8 (9.8175, 4.646) -> (-0.1825, 4.646)
  line L9 (-0.1825, 4.646) -> (-0.1825, -5.354)
  line L10 (-0.1825, -5.354) -> (9.8175, -5.354)
  line L11 (9.8175, -5.354) -> (9.8175, 4.646)
  line L12 (-0.1825, -5.354) -> (-10.1825, -5.354)
  line L13 (-10.1825, -5.354) -> (-10.1825, -15.354)
  line L14 (-10.1825, -15.354) -> (-0.1825, -15.354)
  line L15 (-0.1825, -15.354) -> (-0.1825, -5.354)
  line L16 (-20.5707, -15.354) -> (19.4293, -15.354)
  line L17 (19.4293, -15.354) -> (19.4293, -25.354)
  line L18 (19.4293, -25.354) -> (-20.5707, -25.354)
  line L19 (-20.5707, -25.354) -> (-20.5707, -15.354)
  dimension "d193" = 40
  dimension "d194" = 10
  dimension "d195" = 10
  dimension "d196" = 10
  dimension "d197" = 10
  dimension "d198" = 10
  dimension "d199" = 10
  dimension "d200" = 10
  dimension "d201" = 40
  dimension "d202" = 10
  constraint horizontal L0
  constraint vertical L1
  constraint horizontal L2
  constraint vertical L3
  constraint horizontal L4
  constraint vertical L5
  constraint horizontal L6
  constraint vertical L7
  constraint horizontal L8
  constraint vertical L9
  constraint horizontal L10
  constraint vertical L11
  constraint horizontal L12
  constraint vertical L13
  constraint horizontal L14
  constraint vertical L15
  constraint horizontal L16
  constraint vertical L17
  constraint horizontal L18
  constraint vertical L19
  measures "d193" distance of L0.start L0.end
  measures "d194" distance of L0.start L2.end
  measures "d195" distance of L1.end L4.end
  measures "d196" distance of L1.end L6.end
  measures "d197" distance of L5.end L8.end
  measures "d198" distance of L5.end L10.end
  measures "d199" distance of L9.end L12.end
  measures "d200" distance of L9.end L14.end
  measures "d201" distance of L16.start L16.end
  measures "d202" distance of L16.start L18.end
sketch "Sketch67" plane through (150, 0, 0) normal (1, 0, 0) x (0, 1, 0)
sketch "Sketch68" plane through (-150, 0, 55) normal (-1, 0, 0) x (0, -1, 0)
  line L0 (-100, 10) -> (-70, 10)
  line L1 (-70, 10) -> (-70, -10)
  line L2 (-70, -10) -> (-100, -10)
  line L3 (-100, -10) -> (-100, 10)
  line L4 (90, 10) -> (60, 10)
  line L5 (60, 10) -> (60, -10)
  line L6 (60, -10) -> (90, -10)
  line L7 (90, -10) -> (90, 10)
  constraint horizontal L0
  constraint vertical L1
  constraint horizontal L2
  constraint vertical L3
  constraint horizontal L4
  constraint vertical L5
  constraint horizontal L6
  constraint vertical L7
extrude "Extrude54" add sketch "Sketch62" along normal blind 10 contours L0 L1 L2 L3 L4 L5 L6 L7 L8 L9 L10 L11 bodies 1
sketch "Sketch69" plane through (150, 0, 0) normal (1, 0, 0) x (0, 1, 0)
  line L0 (-80, 25.2282) -> (-80, 50)
  line L1 (-80, 50) -> (-90, 50)
  line L2 (-90, 50) -> (-90, 80)
  line L3 (-90, 80) -> (-80, 80)
  line L4 (-80, 80) -> (-80, 60)
  line L5 (-80, 60) -> (-70, 60)
  line L6 (-70, 60) -> (-70, 80)
  line L7 (-70, 80) -> (-60, 80)
  line L8 (-60, 80) -> (-60, 50)
  line L9 (-60, 50) -> (-70, 50)
  line L10 (-70, 50) -> (-70, 25.2282)
  line L11 (-70, 25.2282) -> (-80, 25.2282)
  line L12 (-100, 25) -> (110, 25)
  line L13 (110, 25) -> (110, 85)
  line L14 (110, 85) -> (-100, 85)
  line L15 (-100, 85) -> (-100, 25)
  line L16 (70, 80) -> (80, 80)
  line L17 (80, 80) -> (80, 30)
  line L18 (80, 30) -> (70, 30)
  line L19 (70, 30) -> (70, 80)
  line L20 (80, 40) -> (90, 40)
  line L21 (90, 40) -> (90, 30)
  line L22 (90, 30) -> (80, 30)
  line L23 (80, 30) -> (80, 40)
  line L24 (90, 80) -> (100, 80)
  line L25 (100, 80) -> (100, 30)
  line L26 (100, 30) -> (90, 30)
  line L27 (90, 30) -> (90, 80)
  constraint horizontal L16
  constraint vertical L17
  constraint horizontal L18
  constraint vertical L19
  constraint horizontal L20
  constraint vertical L21
  constraint horizontal L22
  constraint vertical L23
  constraint coincident L17 L20.start
  constraint horizontal L24
  constraint vertical L25
  constraint horizontal L26
  constraint vertical L27
extrude "Extrude55" add sketch "Sketch69" along normal blind 10 contours L16 L17 L18 L19 L23 | L17 L20 L21 L22 L23 L27 | L21 L24 L25 L26 L27 bodies 1
sketch "Sketch70" plane through (150, 0, 0) normal (1, 0, 0) x (0, 1, 0)
  line L0 (80, 40) -> (90, 40)
  line L1 (90, 40) -> (90, 80)
  line L2 (90, 80) -> (100, 80)
  line L3 (100, 80) -> (100, 30)
  line L4 (100, 30) -> (70, 30)
  line L5 (70, 30) -> (70, 80)
  line L6 (70, 80) -> (80, 80)
  line L7 (80, 80) -> (80, 40)
  line L8 (-80, 25.2282) -> (-80, 50)
  line L9 (-80, 50) -> (-90, 50)
  line L10 (-90, 50) -> (-90, 80)
  line L11 (-90, 80) -> (-80, 80)
  line L12 (-80, 80) -> (-80, 60)
  line L13 (-80, 60) -> (-70, 60)
  line L14 (-70, 60) -> (-70, 80)
  line L15 (-70, 80) -> (-60, 80)
  line L16 (-60, 80) -> (-60, 50)
  line L17 (-60, 50) -> (-70, 50)
  line L18 (-70, 50) -> (-70, 25.2282)
  line L19 (-70, 25.2282) -> (-80, 25.2282)
  line L20 (-100, 25) -> (110, 25)
  line L21 (110, 25) -> (110, 85)
  line L22 (110, 85) -> (-100, 85)
  line L23 (-100, 85) -> (-100, 25)
  line L24 (-20, 80) -> (20, 80)
  line L25 (20, 80) -> (20, 70)
  line L26 (20, 70) -> (-20, 70)
  line L27 (-20, 70) -> (-20, 80)
  line L28 (20, 70) -> (10, 70)
  line L29 (10, 70) -> (10, 60)
  line L30 (10, 60) -> (20, 60)
  line L31 (20, 60) -> (20, 70)
  line L32 (10, 60) -> (0, 60)
  line L33 (0, 60) -> (0, 50)
  line L34 (0, 50) -> (10, 50)
  line L35 (10, 50) -> (10, 60)
  line L36 (0, 50) -> (-10, 50)
  line L37 (-10, 50) -> (-10, 40)
  line L38 (-10, 40) -> (0, 40)
  line L39 (0, 40) -> (0, 50)
  line L40 (-20, 40) -> (20, 40)
  line L41 (20, 40) -> (20, 30)
  line L42 (20, 30) -> (-20, 30)
  line L43 (-20, 30) -> (-20, 40)
  constraint horizontal L24
  constraint vertical L25
  constraint horizontal L26
  constraint vertical L27
  constraint horizontal L28
  constraint vertical L29
  constraint horizontal L30
  constraint vertical L31
  constraint horizontal L32
  constraint vertical L33
  constraint horizontal L34
  constraint vertical L35
  constraint horizontal L36
  constraint vertical L37
  constraint horizontal L38
  constraint vertical L39
  constraint horizontal L40
  constraint vertical L41
  constraint horizontal L42
  constraint vertical L43
extrude "Extrude56" add sketch "Sketch70" along normal blind 10 contours L36 L37 L38 L39 L40 | L32 L33 L34 L35 | L24 L25 L26 L27 L28 | L26 L28 L29 L30 L31 | L38 L40 L41 L42 L43 bodies 1
sketch "Sketch71" plane through (0, 0, 85) normal (0, 0, 1) x (-1, 0, 0)
  line L0 (-110, 90) -> (-100, 90)
  line L1 (-100, 90) -> (-100, 80)
  line L2 (-100, 80) -> (-110, 80)
  line L3 (-110, 80) -> (-110, 90)
  constraint horizontal L0
  constraint vertical L1
  constraint horizontal L2
  constraint vertical L3
extrude "Extrude57" add sketch "Sketch71" along normal blind 50 bodies 1
sketch "Sketch72" plane through (0, 0, 85) normal (0, 0, 1) x (-1, 0, 0)
sketch "Sketch73" plane through (0, 0, 85) normal (0, 0, 1) x (1, 0, 0)
  line L0 (110, -75) -> (100, -75)
  line L1 (100, -75) -> (100, -65)
  line L2 (100, -65) -> (110, -65)
  line L3 (110, -65) -> (110, -75)
  constraint horizontal L0
  constraint vertical L1
  constraint horizontal L2
  constraint vertical L3
extrude "Extrude58" add sketch "Sketch73" along normal blind 50 bodies 1
sketch "Sketch74" plane through (0, 0, 85) normal (0, 0, 1) x (-1, 0, 0)
  line L0 (-110, 60) -> (-100, 60)
  line L1 (-100, 60) -> (-100, 30)
  line L2 (-100, 30) -> (-110, 30)
  line L3 (-110, 30) -> (-110, 60)
  constraint horizontal L0
  constraint vertical L1
  constraint horizontal L2
  constraint vertical L3
extrude "Extrude59" add sketch "Sketch74" along normal blind 10 bodies 1
sketch "Sketch75" plane through (0, 0, 95) normal (0, 0, 1) x (-1, 0, 0)
  line L0 (-110, 30) -> (-100, 30)
  line L1 (-100, 30) -> (-100, 60)
  line L2 (-100, 60) -> (-110, 60)
  line L3 (-110, 60) -> (-110, 30)
  line L4 (-100, 30) -> (-110, 30)
  line L5 (-110, 30) -> (-110, 40)
  line L6 (-110, 40) -> (-100, 40)
  line L7 (-100, 40) -> (-100, 30)
  line L8 (-100, 50) -> (-110, 50)
  line L9 (-110, 50) -> (-110, 60)
  line L10 (-110, 60) -> (-100, 60)
  line L11 (-100, 60) -> (-100, 50)
  constraint horizontal L4
  constraint vertical L5
  constraint horizontal L6
  constraint vertical L7
  constraint coincident L3 L5.end
  constraint coincident L0.end L1.start
  constraint horizontal L8
  constraint vertical L9
  constraint horizontal L10
  constraint vertical L11
  constraint coincident L1 L8.start
extrude "Extrude60" add sketch "Sketch75" along normal blind 40 contours L0 L1 L3 L4 L5 L6 L7 | L1 L2 L3 L8 L9 L10 L11 bodies 1
sketch "Sketch76" plane through (0, -50, 0) normal (0, 1, 0) x (-1, 0, 0)
  line L0 (-110, 95) -> (-100, 95)
  line L1 (-100, 95) -> (-100, 135)
  line L2 (-100, 135) -> (-110, 135)
  line L3 (-110, 135) -> (-110, 95)
sketch "Sketch77" plane through (105, -50, 115) normal (0, 1, 0) x (-1, 0, 0)
sketch "Sketch78" plane through (105, -50, 115) normal (0, 1, 0) x (-1, 0, 0)
  line L0 (-5, 20) -> (5, 20)
  line L1 (5, 20) -> (5, 10)
  line L2 (5, 10) -> (-5, 10)
  line L3 (-5, 10) -> (-5, 20)
  dimension "d253" = 10
  dimension "d254" = 10
  constraint horizontal L0
  constraint vertical L1
  constraint horizontal L2
  constraint vertical L3
  measures "d253" distance of L0.start L0.end
  measures "d254" distance of L0.start L2.end
extrude "Extrude61" add sketch "Sketch78" along normal blind 10 bodies 1
sketch "Sketch79" plane through (0, 0, 85) normal (0, 0, 1) x (1, 0, 0)
  line L0 (110, -20) -> (100, -20)
  line L1 (100, -20) -> (100, 10)
  line L2 (100, 10) -> (110, 10)
  line L3 (110, 10) -> (110, -20)
  constraint horizontal L0
  constraint vertical L1
  constraint horizontal L2
  constraint vertical L3
extrude "Extrude62" add sketch "Sketch79" along normal blind 10 bodies 1